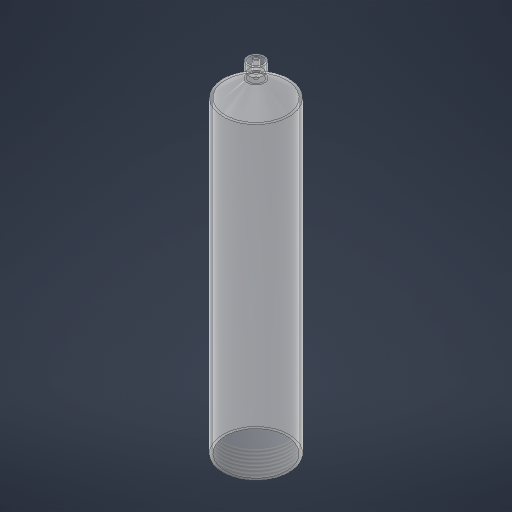
# Autodesk Inventor part: xilanh
Saved by Autodesk Inventor 2027 (Build 310192060, 192F)
## iProperties
Created: 2026-08-20
Part Number: xilanh
Material: PMMA Plastic
Document SubType Name: Modeling
Designer: trtrn
Density: 1.188 g/cm^3
Appearance: Polycarbonate - Clear
Author: trtrn
Autodesk Inventor part; units mm, degrees
ref_plane "YZ Plane" through (0, 0, 0) normal (1, 0, 0) x (0, 1, 0)
ref_plane "XZ Plane" through (0, 0, 0) normal (0, 1, 0) x (-1, 0, 0)
sketch "Sketch1" plane through (0, 0, 0) normal (0, 1, 0) x (-1, 0, 0)
  circle A0 centre (0, 0) radius 19.5
  circle A1 centre (0, 0) radius 18
  dimension "d0" = 39
  dimension "d1" = 36
  constraints: 2 centre point, 2 coincident
  measures "d0" diameter of A0
  measures "d1" diameter of A1
extrude "Extrusion1" add sketch "Sketch1" along normal blind 182
ref_plane "Work Plane1" through (0, 192, 0) normal (0, 1, 0) x (1, 0, 0)
sketch "Sketch2" plane through (0, 192, 0) normal (0, 1, 0) x (1, 0, 0)
  circle A0 centre (0, 0) radius 5
  dimension "d5" = 10
  constraints: 1 centre point, 1 coincident
  measures "d5" diameter of A0
loft "Loft1" add profiles "Sketch2" section 1 edges at (19.5, 182, 0)
sketch "Sketch3" plane through (0, 192, 0) normal (0, 1, 0) x (1, 0, 0)
  circle A0 centre (0, 0) radius 4
  dimension "d11" = 8
  constraints: 1 centre point, 1 coincident
  measures "d11" diameter of A0
loft "Loft2" cut profiles "Sketch3" section 1 edges at (18, 182, 0)
sketch "Sketch4" plane through (0, 192, 0) normal (0, 1, 0) x (1, 0, 0)
  circle A0 centre (0, 0) radius 5
  circle A1 centre (0, 0) radius 4
  circle A2 centre (0, 0) radius 5 projected
  dimension "d16" = 10
  dimension "d17" = 8
  constraints: 2 centre point, 1 coincident, 1 concentric
  measures "d16" diameter of A0
  measures "d17" diameter of A1
extrude "Extrusion2" add sketch "Sketch4" along normal blind 9
sketch "Sketch5" plane through (0, 192, 0) normal (0, 1, 0) x (1, 0, 0)
  circle A0 centre (0, 0) radius 4
  circle A1 centre (0, 0) radius 4 projected
  constraints: 1 centre point, 1 coincident, 1 concentric
ref_plane "Work Plane2" through (0, 202, 0) normal (0, 1, 0) x (1, 0, 0)
sketch "Sketch6" plane through (0, 202, 0) normal (0, 1, 0) x (1, 0, 0)
  circle A0 centre (0, 0) radius 1.5
  line L0 (1.5, 0) -> (-1.5, 0) construction
  dimension "d21" = 3
  constraints: 2 end point, 2 point on circle, 1 centre point, 1 coincident, 1 horizontal, 1 midpoint
  measures "d21" diameter of A0
extrude "Extrusion3" add sketch "Sketch5" along normal blind 3
extrude "Extrusion4" add sketch "Sketch6" against normal up to surface (7 mm away)
sketch "Sketch8" plane through (0, 202, 0) normal (0, 1, 0) x (1, 0, 0)
  circle A0 centre (0, 0) radius 1.5 projected
  circle A1 centre (0, 0) radius 1
  dimension "d26" = 2
  constraints: 1 centre point, 1 coincident
  measures "d26" diameter of A1
extrude "Extrusion5" cut sketch "Sketch8" against normal through all contours A1
thread "Thread1" size "M39x2" class "6g" standard "ANSI Metric M Profile" length 16
body "Solid1"
